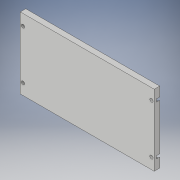
# Autodesk Inventor part: front
Saved by Autodesk Inventor 2017 (Build 210142000, 142)
## iProperties
Created: 2016-07-21
Part Number: front
Material: Generic
Document SubType Name: Modeling
Designer: Darien Morrow
Density: 1 g/cm^3
Appearance: Default
Author: Darien Morrow
Autodesk Inventor part; units mm, degrees
ref_plane "YZ Plane" through (0, 0, 0) normal (1, 0, 0) x (0, 1, 0)
ref_plane "XZ Plane" through (0, 0, 0) normal (0, 1, 0) x (-1, 0, 0)
ref_plane "XY Plane" through (0, 0, 0) normal (0, 0, 1) x (1, 0, 0)
sketch "Sketch1" plane through (0, 0, 0) normal (0, 0, 1) x (1, 0, 0)
  line L0 (-77.7875, -41.275) -> (77.7875, -41.275)
  line L1 (77.7875, -41.275) -> (77.7875, 41.275)
  line L2 (77.7875, 41.275) -> (-77.7875, 41.275)
  line L3 (-77.7875, 41.275) -> (-77.7875, -41.275)
  line L4 (-77.7875, -41.275) -> (77.7875, 41.275) construction
  line L5 (77.7875, -41.275) -> (-77.7875, 41.275) construction
  point P0 (0, 0)
  dimension "d0" = 155.575
  dimension "d1" = 82.55
  constraints: 12 end point, 2 midpoint, 2 parallel, 1 horizontal, 1 perpendicular
  measures "d0" distance of L2.end L1.end
  measures "d1" distance between parallel lines of L0 L2
extrude "Extrusion1" add sketch "Sketch1" along normal blind 6.35
sketch "Sketch2" plane through (0, 0, 0) normal (0, 0, -1) x (-1, 0, 0)
  line L0 (-74.6125, -28.575) -> (74.6125, -28.575)
  line L1 (74.6125, -28.575) -> (74.6125, 28.575)
  line L2 (74.6125, 28.575) -> (-74.6125, 28.575)
  line L3 (-74.6125, 28.575) -> (-74.6125, -28.575)
  line L4 (-74.6125, -28.575) -> (74.6125, 28.575) construction
  line L5 (74.6125, -28.575) -> (-74.6125, 28.575) construction
  point P0 (0, 0)
  dimension "d4" = 149.225
  dimension "d5" = 57.15
  constraints: 12 end point, 4 coincident, 2 midpoint, 2 parallel, 1 horizontal, 1 perpendicular
  measures "d4" distance of L2.end L1.end
  measures "d5" distance between parallel lines of L0 L2
hole "Hole1" at (74.6125, 28.575, 0) at (74.6125, -28.575, 0) at (-74.6125, 28.575, 0) at (-74.6125, -28.575, 0) direction (0, 0, 1) diameter 3.81 end through all counterbore diameter 7.1374 counterbore depth 3.5052 clearance for "Socket Head Cap Screw" size "#6" standard "Ansi Unified Screw Threads"
body "Solid1"
